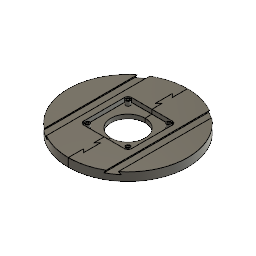
rotatePlate (Autodesk Fusion 360 design; units mm, degrees)
Autodesk Fusion 360 part; units mm, degrees
sketch "Skizze1" plane through (0, 0, 0) normal (0, 1, 0) x (1, 0, 0)
  circle A0 centre (0, 0) radius 70
  dimension "d1" = 140
  measures "d1" diameter of A0
extrude "Extrusion1" add sketch "Skizze1" against normal blind 10 makes body 1
sketch "Skizze2" plane through (0, 0, 0) normal (0, 1, 0) x (-1, 0, 0)
  circle A0 centre (0, 0) radius 70
  circle A1 centre (0, 0) radius 20
  line L0 (-28, -28) -> (28, -28)
  line L1 (28, -28) -> (28, 28)
  line L2 (28, 28) -> (-28, 28)
  line L3 (-28, 28) -> (-28, -28)
  line L4 (-28, -28) -> (28, 28) construction
  line L5 (28, -28) -> (-28, 28) construction
  circle A2 centre (-23.75, -23.75) radius 1.45
  circle A3 centre (23.75, -23.75) radius 1.45
  circle A4 centre (23.75, 23.75) radius 1.45
  circle A5 centre (-23.75, 23.75) radius 1.45
  dimension "d4" = 40
  dimension "d5" = 56
  dimension "d6" = 56
  dimension "d11" = 2.9
  dimension "d12" = 4.25
  dimension "d13" = 2.9
  dimension "d14" = 2.9
  dimension "d15" = 2.9
  dimension "d16" = 4.25
  dimension "d17" = 4.25
  dimension "d18" = 4.25
  measures "d4" diameter of A1
  measures "d11" diameter of A2
  measures "d13" diameter of A3
  measures "d14" diameter of A4
  measures "d15" diameter of A5
extrude "Extrusion2" cut sketch "Skizze2" against normal blind 10 contours A1 bodies 1
extrude "Extrusion3" cut sketch "Skizze2" against normal blind 5 contours L0 L1 L2 L3 | A2 | A3 | A4 | A5 bodies 1
extrude "Extrusion4" cut sketch "Skizze2" against normal blind 10 contours A2 | A3 | A4 | A5 bodies 1
sketch "Skizze3" plane through (0, -5, 0) normal (0, 1, 0) x (-1, 0, 0)
  circle A0 centre (23.75, -23.75) radius 1.45
  circle A1 centre (23.75, 23.75) radius 1.45
  circle A2 centre (-23.75, -23.75) radius 1.45
  circle A3 centre (-23.75, 23.75) radius 1.45
  circle A4 centre (0, 0) radius 20
  line L0 (-28, 28) -> (-28, -28)
  line L1 (-28, -28) -> (28, -28)
  line L2 (28, -28) -> (28, 28)
  line L3 (28, 28) -> (-28, 28)
  circle A5 centre (23.75, 23.75) radius 2.5
  circle A6 centre (-23.75, 23.75) radius 2.5
  circle A7 centre (-23.75, -23.75) radius 2.5
  circle A8 centre (23.75, -23.75) radius 2.5
  dimension "d21" = 5
  dimension "d22" = 5
  dimension "d23" = 5
  dimension "d24" = 5
  measures "d21" diameter of A5
  measures "d22" diameter of A6
  measures "d23" diameter of A7
  measures "d24" diameter of A8
extrude "Extrusion5" add sketch "Skizze3" along normal blind 5 contours A5 | A6 | A7 | A8 bodies 1
sketch "Skizze4" plane through (0, -10, 0) normal (0, -1, 0) x (1, 0, 0)
  circle A0 centre (-23.75, -23.75) radius 1.45
  circle A1 centre (-23.75, 23.75) radius 1.45
  circle A2 centre (23.75, -23.75) radius 1.45
  circle A3 centre (23.75, 23.75) radius 1.45
  circle A4 centre (0, 0) radius 20
  circle A5 centre (0, 0) radius 70
  circle A6 centre (23.75, 23.75) radius 3
  circle A7 centre (-23.75, 23.75) radius 3
  circle A8 centre (-23.75, -23.75) radius 3
  circle A9 centre (23.75, -23.75) radius 3
  dimension "d27" = 6
  dimension "d28" = 6
  dimension "d29" = 6
  dimension "d30" = 6
  measures "d27" diameter of A6
  measures "d28" diameter of A7
  measures "d29" diameter of A8
  measures "d30" diameter of A9
extrude "Extrusion6" cut sketch "Skizze4" against normal blind 2.3 contours A6 | A7 | A8 | A9 bodies 1
fillet "Abrundung1" radius 4 4 edges at (28, -2.5, -28) (-28, -2.5, -28) (28, -2.5, 28) (-28, -2.5, 28) on bodies 1
sketch "Skizze5" plane through (0, 0, 0) normal (0, 0, 1) x (1, 0, 0)
  line L0 (35, 0) -> (33.2679, -3)
  line L1 (33.2679, -3) -> (45.2679, -3)
  line L2 (45.2679, -3) -> (43.5359, 0)
  line L3 (0, 0) -> (0, 30.2338) construction
  line L4 (0, 0) -> (22.4086, 0) construction
  line L5 (43.5359, 0) -> (35, 0)
  line L6 (-43.5359, 0) -> (-35, 0)
  line L7 (-45.2679, -3) -> (-43.5359, 0)
  line L8 (-35, 0) -> (-33.2679, -3)
  line L9 (-33.2679, -3) -> (-45.2679, -3)
  dimension "d34" = 60
  dimension "d35" = 60
  dimension "d36" = 12
  dimension "d37" = 3
  dimension "d38" = 35
  measures "d34" angle of L0 L1
  measures "d35" angle of L1 L2
  measures "d37" distance of L1 L4
extrude "Extrusion7" cut sketch "Skizze5" along normal mid plane 212 bodies 1
sketch "Skizze6" plane through (0, 0, 0) normal (0, 1, 0) x (1, 0, 0)
  arc A0 (35, 60.6218) -> (-35, 60.6218) centre (0, 0) ccw
  arc A1 (-35, -60.6218) -> (35, -60.6218) centre (0, 0) ccw
  line L0 (24, -28) -> (-24, -28)
  line L1 (0, -40) -> (4, -36)
  line L2 (4, -36) -> (4, -56)
  line L3 (4, -56) -> (0, -52)
  arc A2 (43.5359, -54.8145) -> (43.5359, 54.8145) centre (0, 0) ccw construction
  line L4 (-70, 0) -> (70, 0) construction
  line L5 (0, 40) -> (-4, 36)
  line L6 (-4, 36) -> (-4, 56)
  line L7 (-4, 56) -> (0, 52)
  line L8 (0, -70) -> (0, -52)
  line L9 (0, -40) -> (0, 40)
  line L10 (0, 52) -> (0, 70)
  dimension "d44" = 40
  dimension "d45" = 20
  measures "d44" distance of A0.centre
surface "Extrusion8" add extruded along (0, 1, 0) between -29 and 29 path "Skizze6" along L8 L3 L2 L1 L9 L5 L6 L7 L10 separate body makes body 2
split "Teilen1" by bodies 2 bodies 1 makes body 3 at (-17.8181, -10, 47.2475)
hidden bodies 2
equation "d13 = d11"
equation "d14 = d11"
equation "d15 = d11"
equation "d16 = d12"
equation "d17 = d12"
equation "d18 = d12"
equation "d35 = d34"
